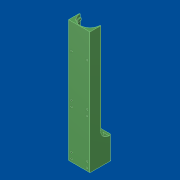
# Autodesk Inventor part: 402-gearbox-housing
Saved by Autodesk Inventor 2018 (Build 220112000, 112)
## iProperties
Created: 2020-06-11
Part Number: 402-gearbox-housing
Material: Generic
Document SubType Name: Modeling
Designer: Bunny320
Density: 1 g/cm^3
Appearance: Smooth - Dark Forest Green
Author: Bunny320
## iProperties of the stored document 402-gearbox-housing_3DPrint.ipt
Created: 2020-06-27
Part Number: 402-gearbox-housing_3DPrint
Material: Generic
Document SubType Name: Modeling
Designer: Bunny320
Density: 1 g/cm^3
Appearance: Default
Author: Bunny320
Autodesk Inventor part; units mm, degrees
ref_plane "YZ Plane" through (0, 0, 0) normal (1, 0, 0) x (0, 1, 0)
ref_plane "XZ Plane" through (0, 0, 0) normal (0, 1, 0) x (-1, 0, 0)
ref_plane "XY Plane" through (0, 0, 0) normal (0, 0, 1) x (1, 0, 0)
sketch "Sketch1" plane through (0, 0, 0) normal (0, 0, 1) x (1, 0, 0)
  line L0 (-19, -19) -> (19, -19)
  line L1 (19, -19) -> (19, 19)
  line L2 (19, 19) -> (-19, 19)
  line L3 (-19, 19) -> (-19, -19)
  line L4 (-19, -19) -> (19, 19) construction
  line L5 (19, -19) -> (-19, 19) construction
  point P0 (0, 0)
  dimension "d0" = 38
  constraints: 12 end point, 2 midpoint, 2 parallel, 2 perpendicular, 1 horizontal
  measures "d0" distance of L1.end L2.end
extrude "Extrusion1" add sketch "Sketch1" along normal blind 217
sketch "Sketch2" plane through (0, 0, 0) normal (0, 0, -1) x (-1, 0, 0)
  circle A0 centre (0, 0) radius 16.1
  dimension "d3" = 32.2
  constraints: 1 centre point, 1 coincident
  measures "d3" diameter of A0
extrude "Extrusion2" cut sketch "Sketch2" against normal blind 32
sketch "Sketch3" plane through (0, 0, 217) normal (0, 0, 1) x (1, 0, 0)
  circle A0 centre (0, 0) radius 17
  dimension "d6" = 34
  constraints: 1 centre point, 1 coincident
  measures "d6" diameter of A0
extrude "Extrusion3" cut sketch "Sketch3" against normal blind 177
sketch "Sketch4" plane through (0, 0, 40) normal (0, 0, 1) x (1, 0, 0)
  circle A0 centre (0, 0) radius 10
  dimension "d9" = 20
  constraints: 1 centre point, 1 coincident
  measures "d9" diameter of A0
extrude "Extrusion4" cut sketch "Sketch4" against normal through all
sketch "Sketch5" plane through (0, 0, 40) normal (0, 0, 1) x (1, 0, 0)
  point P0 (0, 0)
  point P1 (0, 13)
  dimension "d12" = 13
  constraints: 1 vertical alignment
  measures "d12" distance of point (0, 0) point (0, 13)
hole "Hole1" at (0, 13, 40) direction (0, 0, -1) diameter 3.4 end through all countersink diameter 7.5 countersink angle 90 clearance for "Countersunk Flat Head Hex Socket Screw DIN EN ISO 10642" size "M3" standard "DIN"
pattern_circular "Circular Pattern1" count 4 over 360 about axis through (0, 0, -10) along (0, 0, 1) of "Hole1"
sketch "Sketch7" plane through (0, 0, 0) normal (0, 1, 0) x (-1, 0, 0)
  line L0 (17, 78.95) -> (7.4, 78.95)
  line L1 (7.4, 78.95) -> (7.4, 81.95)
  line L2 (7.4, 81.95) -> (8.5, 81.95)
  line L3 (8.5, 81.95) -> (8.5, 88.05)
  line L4 (8.5, 88.05) -> (7.4, 88.05)
  line L5 (7.4, 88.05) -> (7.4, 91.05)
  line L6 (7.4, 91.05) -> (17, 91.05)
  line L7 (17, 217) -> (17, 40) projected
  line L8 (17, 91.05) -> (17, 78.95)
  line L9 (0, 88.2429) -> (0, 190.8877)
  line L10 (0, -42) -> (0, 252) projected
  line L11 (1.9638, 40) -> (9.8053, 40) projected
  line L12 (17, 164.9) -> (7.4, 164.9)
  line L13 (7.4, 164.9) -> (7.4, 167.9)
  line L14 (7.4, 167.9) -> (8.5, 167.9)
  line L15 (8.5, 167.9) -> (8.5, 174)
  line L16 (8.5, 174) -> (7.4, 174)
  line L17 (7.4, 174) -> (7.4, 177)
  line L18 (7.4, 177) -> (17, 177)
  line L19 (17, 177) -> (17, 164.9)
  line L20 (-17, 217) -> (17, 217) projected
  line L21 (17, 212) -> (16, 212)
  line L22 (16, 212) -> (16, 208)
  line L23 (16, 208) -> (17, 208)
  line L24 (17, 208) -> (17, 212)
  line L25 (17, 217) -> (17, 40) projected
  line L26 (-19, 0) -> (19, 0) projected
  point P0 (0, 0)
  point P1 (1, 89.2429)
  dimension "d26" = 17
  dimension "d27" = 14.8
  dimension "d28" = 6.1
  dimension "d29" = 3
  dimension "d34" = 14.8
  dimension "d35" = 17
  dimension "d36" = 3
  dimension "d37" = 40
  dimension "d38" = 6.1
  dimension "d39" = 5
  dimension "d40" = 9
  dimension "d41" = 32
  dimension "d75" = 81.95
  constraints: 42 end point, 14 perpendicular, 8 point on line, 4 collinear, 3 horizontal, 1 vertical
  measures "d26" diameter of L3 L9
  measures "d27" diameter of L1 L9
  measures "d28" distance of L2.end L3.end
  measures "d29" distance of L4.end L5.end
  measures "d34" diameter of L13 L9
  measures "d35" diameter of L15 L9
  measures "d36" distance between parallel lines of L18 L16
  measures "d37" distance between parallel lines of L20 L18
  measures "d38" distance of L14.end L15.end
  measures "d39" distance between parallel lines of L20 L21
  measures "d40" distance between parallel lines of L20 L23
  measures "d41" diameter of L22 L9
  measures "d75" distance from line of L2.end L26
revolve "Revolution1" add sketch "Sketch7" angle 360 about axis through (0, 0, 88.2429) along (0, 0, 1)
sketch "Sketch8" plane through (0, 0, 217) normal (0, 0, 1) x (1, 0, 0)
  circle A0 centre (0, 0) radius 17.75
  dimension "d42" = 35.5
  constraints: 1 centre point, 1 coincident
  measures "d42" diameter of A0
extrude "Extrusion6" cut sketch "Sketch8" against normal up to surface (5 mm away)
sketch "Sketch10" plane through (-19, -19, 0) normal (0, -1, 0) x (1, 0, 0)
  line L0 (33, 170.95) -> (5, 170.95)
  line L1 (5, 170.95) -> (5, 85)
  line L2 (5, 85) -> (33, 85)
  line L3 (33, 85) -> (33, 170.95)
  line L4 (11.6, 174) -> (26.4, 174) projected
  line L5 (11.6, 81.95) -> (26.4, 81.95) projected
  line L6 (0, 0) -> (0, 217) projected
  line L7 (38, 0) -> (38, 217) projected
  point P0 (19, 0)
  dimension "d56" = 3.05
  dimension "d57" = 3.05
  dimension "d58" = 5
  dimension "d59" = 5
  constraints: 8 end point, 4 coincident, 2 parallel, 1 horizontal, 1 perpendicular
  measures "d56" distance between parallel lines of L4 L0
  measures "d57" distance between parallel lines of L5 L2
  measures "d58" distance between parallel lines of L6 L1
  measures "d59" distance between parallel lines of L7 L3
hole "Hole3" at (-14, -19, 170.95) at (14, -19, 170.95) at (14, -19, 85) at (-14, -19, 85) direction (0, 1, 0) diameter 2.459 end through all thread size "M3x0.5" class "6H" standard "ISO Metric profile"
sketch "Sketch11" plane through (0, 0, 217) normal (0, 0, 1) x (1, 0, 0)
  line L0 (19, 19) -> (-19, 19) projected
  line L1 (19, -19) -> (19, 19) projected
  line L2 (-19, 19) -> (19, 19)
  line L3 (19, 19) -> (19, 0)
  line L4 (19, 0) -> (-19, 0)
  line L5 (-19, 0) -> (-19, 19)
  point P0 (0, 0)
  constraints: 8 end point, 2 parallel, 1 horizontal, 1 midpoint, 1 perpendicular
extrude "Extrusion7" cut sketch "Sketch11" against normal up to surface (177 mm away)
sketch "Sketch12" plane through (-19, -19, 0) normal (0, -1, 0) x (1, 0, 0)
  line L0 (5, 5) -> (33, 5)
  line L1 (33, 5) -> (33, 15)
  line L2 (33, 15) -> (5, 15)
  line L3 (5, 15) -> (5, 5)
  line L4 (5, 85) -> (33, 85)
  line L5 (33, 85) -> (33, 95)
  line L6 (33, 95) -> (5, 95)
  line L7 (5, 95) -> (5, 85)
  line L8 (0, 0) -> (0, 217) projected
  line L9 (0, 0) -> (38, 0) projected
  line L10 (38, 0) -> (38, 217) projected
  point P0 (19, 0)
  dimension "d69" = 5
  dimension "d70" = 5
  dimension "d71" = 5
  dimension "d72" = 10
  dimension "d73" = 10
  dimension "d74" = 85
  constraints: 16 end point, 6 coincident, 4 parallel, 2 horizontal, 2 perpendicular, 2 point on line
  measures "d69" distance between parallel lines of L8 L3
  measures "d70" distance between parallel lines of L9 L0
  measures "d71" distance between parallel lines of L10 L1
  measures "d72" distance of L0.end L1.end
  measures "d73" distance of L4.end L5.end
  measures "d74" distance between parallel lines of L9 L4
hole "Hole4" at (-14, -19, 5) at (-14, -19, 15) at (14, -19, 5) at (14, -19, 15) at (-14, -19, 95) at (14, -19, 95) direction (0, 1, 0) diameter 2.459 depth 16 tip angle 118 thread size "M3x0.5" class "6H" standard "ISO Metric profile"
fillet "Fillet1" radius 15 2 edges at (-18, 0, 40) (18, 0, 40)
fillet "Fillet2" radius 2 2 edges at (19, 19, 20) (-19, 19, 20)
equation "\"d34\" = d27"
equation "\"d35\" = d26"
equation "\"d36\" = d29"
equation "\"d37\" = d30"
equation "\"d38\" = d28"
equation "\"d56\" = 0.5 * d28"
equation "\"d57\" = d56"
equation "\"d59\" = d58"
equation "\"d70\" = d69"
equation "\"d71\" = d69"
equation "\"d73\" = d72"
equation "\"d30\" = 40"
body "Solid1"
